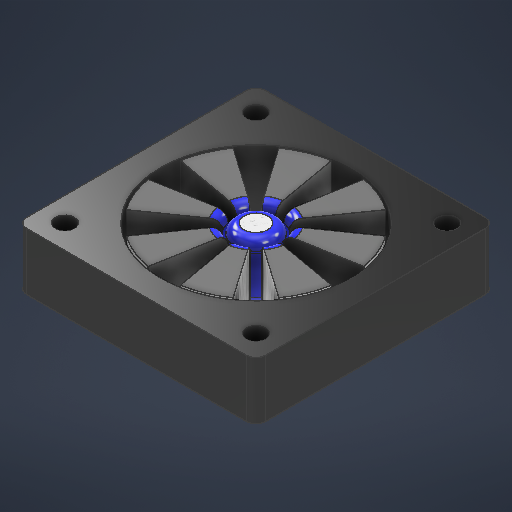
# Autodesk Inventor part: bigbuckfan
Saved by Autodesk Inventor 2026.1 (Build 301233000, 233)
## iProperties
Created: 2026-04-26
Part Number: bigbuckfan
Material: Generic
Document SubType Name: Modeling
Designer: emanuel
Density: 1 g/cm^3
Appearance: Default
Author: emanuel
Autodesk Inventor part; units mm, degrees
ref_plane "YZ Plane" through (0, 0, 0) normal (1, 0, 0) x (0, 1, 0)
ref_plane "XZ Plane" through (0, 0, 0) normal (0, 1, 0) x (-1, 0, 0)
ref_plane "XY Plane" through (0, 0, 0) normal (0, 0, 1) x (1, 0, 0)
sketch "Sketch1" plane through (0, 0, 0) normal (0, 1, 0) x (-1, 0, 0)
  line L0 (0, 0) -> (50, 0)
  line L1 (50, 0) -> (50, -50)
  line L2 (50, -50) -> (0, -50)
  line L3 (0, -50) -> (0, 0)
  dimension "d0" = 50
  dimension "d1" = 50
  constraints: 8 end point, 2 parallel, 1 horizontal, 1 perpendicular
  measures "d0" distance of L1.end L2.end
  measures "d1" distance of L0.end L1.end
extrude "Extrusion1" add sketch "Sketch1" along normal blind 12
fillet "Fillet1" radius 2 4 edges at (-50, 6, 0) (0, 6, 0) (0, 6, -50) (-50, 6, -50)
sketch "Sketch2" plane through (0, 12, 0) normal (0, 1, 0) x (1, 0, 0)
  line L0 (-50, 50) -> (-25, 50)
  line L1 (-25, 50) -> (-25, 25)
  line L2 (-25, 25) -> (-50, 25)
  line L3 (-50, 25) -> (-50, 50)
  circle A0 centre (-25, 25) radius 20
  circle A1 centre (-25, 25) radius 5
  line L4 (-25, 25) -> (-28.473, 44.6962)
  line L5 (-25, 25) -> (-5, 25) construction
  line L6 (-25, 25) -> (-21.527, 44.6962)
  line L7 (-25, 25) -> (-5, 25) construction
  line L8 (-25, 25) -> (-41.383, 36.4715)
  line L9 (-25, 25) -> (-36.4715, 41.383)
  line L10 (-25, 25) -> (-44.6962, 21.527)
  line L11 (-25, 25) -> (-44.6962, 28.473)
  line L12 (-25, 25) -> (-36.4715, 8.617)
  line L13 (-25, 25) -> (-41.383, 13.5285)
  line L14 (-25, 25) -> (-21.527, 5.3038)
  line L15 (-25, 25) -> (-28.473, 5.3038)
  line L16 (-25, 25) -> (-8.617, 13.5285)
  line L17 (-25, 25) -> (-13.5285, 8.617)
  line L18 (-25, 25) -> (-5.3038, 28.473)
  line L19 (-25, 25) -> (-5.3038, 21.527)
  line L20 (-25, 25) -> (-13.5285, 41.383)
  line L21 (-25, 25) -> (-8.617, 36.4715)
  point P0 (0, 0)
  point P1 (-27.8679, 29.0958)
  point P2 (-29.0958, 27.8679)
  point P3 (-24.1318, 29.924)
  point P4 (-25.8682, 29.924)
  point P5 (-20.9042, 27.8679)
  point P6 (-22.1321, 29.0958)
  point P7 (-20.076, 24.1318)
  point P8 (-20.076, 25.8682)
  point P9 (-22.1321, 20.9042)
  point P10 (-20.9042, 22.1321)
  point P11 (-25.8682, 20.076)
  point P12 (-24.1318, 20.076)
  point P13 (-29.0958, 22.1321)
  point P14 (-27.8679, 20.9042)
  point P15 (-29.924, 24.1318)
  point P16 (-29.924, 25.8682)
  dimension "d5" = 25
  dimension "d6" = 25
  dimension "d7" = 40
  dimension "d8" = 10
  dimension "d9" = 100
  dimension "d10" = 80
  dimension "d13" = 360
  constraints: 44 end point, 3 horizontal, 2 centre point, 2 coincident, 2 equal length, 2 parallel, 2 point on circle, 1 perpendicular, 41 other
  measures "d5" distance of L1.end L2.end
  measures "d6" distance of L0.end L1.end
  measures "d7" diameter of A0
  measures "d8" diameter of A1
  measures "d9" angle of L5 L4
  measures "d10" angle of L7 L6
extrude "Extrusion2" cut sketch "Sketch2" against normal blind 12 contours A0 L6 A1 L1 | L1 A1 L4 A0 | A0 L11 A1 L2 | L2 A1 L10 A0 | A0 L21 A1 L20 | L9 A1 L8 A0 | L13 A1 L12 A0 | L14 A0 L15 A1 | L16 A0 L17 A1 | L18 A0 L19 A1
sketch "Sketch3" plane through (0, 12, 0) normal (0, 1, 0) x (1, 0, 0)
  arc A0 (-27.8679, 29.0958) -> (-29.0958, 27.8679) centre (-25, 25) ccw projected
  circle A1 centre (-25, 25) radius 5
  circle A2 centre (-25, 25) radius 4.5
  point P0 (0, 0)
  dimension "d17" = 9
  constraints: 2 coincident, 1 centre point, 3 other
  measures "d17" diameter of A2
extrude "Extrusion3" cut sketch "Sketch3" against normal blind 2
fillet "Fillet2" radius 2 9 edges at (-29.5, 12, -25) (-29.6194, 12, -23.0866) (-29.6194, 12, -26.9134) (-26.9134, 12, -29.6194) (-23.0866, 12, -29.6194) (-20.3806, 12, -26.9134) (-20.3806, 12, -23.0866) (-23.0866, 12, -20.3806) (-26.9134, 12, -20.3806)
sketch "Sketch4" plane through (0, 12, 0) normal (0, 1, 0) x (1, 0, 0)
  line L0 (-50, 50) -> (-45, 50)
  line L1 (-45, 50) -> (-45, 45)
  line L2 (-45, 45) -> (-50, 45)
  line L3 (-50, 45) -> (-50, 50)
  line L4 (-45, 45) -> (-5, 45)
  line L5 (-5, 45) -> (-5, 5)
  line L6 (-5, 5) -> (-45, 5)
  line L7 (-45, 5) -> (-45, 45)
  circle A0 centre (-45, 5) radius 2
  circle A1 centre (-45, 45) radius 2
  circle A2 centre (-5, 45) radius 2
  circle A3 centre (-5, 5) radius 2
  point P0 (0, 0)
  dimension "d21" = 5
  dimension "d22" = 5
  dimension "d23" = 40
  dimension "d24" = 40
  dimension "d25" = 4
  dimension "d26" = 4
  dimension "d27" = 4
  dimension "d28" = 4
  constraints: 16 end point, 4 centre point, 4 coincident, 4 parallel, 2 horizontal, 2 perpendicular
  measures "d21" distance of L1.end L2.end
  measures "d22" distance of L0.end L1.end
  measures "d23" distance of L5.end L6.end
  measures "d24" distance of L4.end L5.end
  measures "d25" diameter of A0
  measures "d26" diameter of A1
  measures "d27" diameter of A2
  measures "d28" diameter of A3
extrude "Extrusion4" cut sketch "Sketch4" against normal blind 12 contours A1 L4 L1 | L1 L2 A1 | L2 L7 A1 | L4 A1 L7 | A2 L5 L4 | L4 L5 A2 | A0 L6 L7 | L7 L6 A0 | A3 L6 L5 | L5 L6 A3
sketch "Sketch5" plane through (0, 0, 0) normal (0, -1, 0) x (1, 0, 0)
  arc A0 (-29.924, -24.1318) -> (-29.924, -25.8682) centre (-25, -25) ccw projected
  circle A1 centre (-25, -25) radius 5
  circle A2 centre (-25, -25) radius 4.5
  point P0 (0, 0)
  dimension "d31" = 9
  constraints: 2 coincident, 1 centre point, 3 other
  measures "d31" diameter of A2
extrude "Extrusion5" cut sketch "Sketch5" against normal blind 2
fillet "Fillet3" radius 2 9 edges at (-29.5, 0, -25) (-29.6194, 0, -26.9134) (-26.9134, 0, -29.6194) (-23.0866, 0, -29.6194) (-29.6194, 0, -23.0866) (-26.9134, 0, -20.3806) (-23.0866, 0, -20.3806) (-20.3806, 0, -23.0866) (-20.3806, 0, -26.9134)
sketch "Sketch7" plane through (0, 12, 0) normal (0, 1, 0) x (1, 0, 0)
  circle A0 centre (-25, 25) radius 2.5 projected
  arc A1 (-8.617, 36.4715) -> (-13.5285, 41.383) centre (-25, 25) ccw projected
  circle A2 centre (-25, 25) radius 20
  circle A3 centre (-25, 25) radius 19.5
  point P0 (0, 0)
  point P1 (-13.5285, 41.383)
  dimension "d38" = 39
  constraints: 2 coincident, 1 centre point, 3 other
  measures "d38" diameter of A3
extrude "Extrusion7" cut sketch "Sketch7" against normal blind 12 contours A2 A1
body "Solid1"
